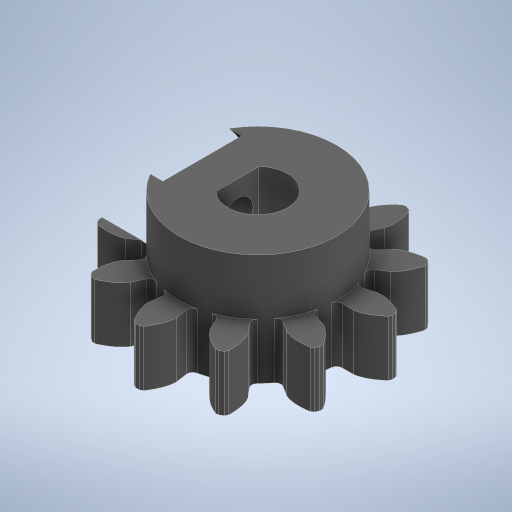
# Autodesk Inventor part: screw_gear_under_12
Saved by Autodesk Inventor 2024.1 (Build 281209000, 209)
## iProperties
Created: 2025-01-10
Part Number: screw_gear_under_12
Material: 一般
Document SubType Name: Modeling
Designer: hibik
Density: 1 g/cm^3
Appearance: 既定
Author: hibik
Autodesk Inventor part; units mm, degrees
ref_plane "XZ Plane" through (0, 0, 0) normal (0, 1, 0) x (-1, 0, 0)
ref_plane "XY Plane" through (0, 0, 0) normal (0, 0, 1) x (1, 0, 0)
sketch "スケッチ1" plane through (0, 0, 0) normal (0, 1, 0) x (-1, 0, 0)
  circle A0 centre (0, 0) radius 5.5 construction
  circle A1 centre (0, 0) radius 5.1683 construction
  line L0 (0, 0) -> (0.7355, -5.1157)
  line L1 (0, -10.5007) -> (0, 8.7501) projected
  dimension "d1" = 10.3366
  dimension "d0" = 11
  dimension "d4" = 8.182
  constraints: 3 coincident, 2 end point, 1 centre point, 7 other
  measures "d0" diameter of A0
  measures "d4" angle of L1 L0
sketch "スケッチ2" plane through (0, 0, 0) normal (0, 1, 0) x (-1, 0, 0)
  circle A0 centre (0, 0) radius 6.5
  dimension "d5" = 13
  constraints: 1 centre point, 1 coincident
  measures "d5" diameter of A0
extrude "押し出し1" add sketch "スケッチ2" along normal blind 3
sketch "スケッチ3" plane through (0, 3, 0) normal (0, 1, 0) x (1, 0, 0)
  line L0 (0, 0) -> (-0.7355, 5.1157) projected
  spline S0 degree 3 poles (-0.7355, 5.1157) (-0.7355, 5.1158) (-0.8126, 5.5427) (-1.3851, 6.0793) (-1.6608, 6.3379) (-2.0474, 6.6147) (-2.557, 6.8472) knots 0 0 0 0 0.674859 0.674859 0.674859 1 1 1 1 projected
  circle A0 centre (0, 0) radius 6.5 projected
  circle A1 centre (0, 0) radius 4.25
  line L1 (0, 10.7) -> (0, -9.95) projected
  point P0 (0, 4.25)
  point P1 (0, 6.5)
  point P2 (-1.6329, 6.2915)
  point P3 (-0.6048, 4.2067)
  dimension "d10" = 8.5
  constraints: 3 coincident, 1 centre point
  measures "d10" diameter of A1
extrude "押し出し2" cut sketch "スケッチ3" against normal through all contours L0 S0 A0 L1 A1 picked at (-0.2452, 5.2886)
fillet "フィレット1" radius 0.3 1 edges at (-0.6048, 1.5, -4.2067)
chamfer "面取り1" distance 0.1 angle 45 1 edges at (-1.6329, 1.5, -6.2915)
mirror "ミラー1" about plane through (0, 3, -6.5) normal (-1, 0, 0) of "押し出し2", "フィレット1", "面取り1"
pattern_circular "円形状パターン1" count 11 over 360 about axis through (0, -10, 0) along (0, 1, 0) of "押し出し2", "フィレット1", "面取り1", "ミラー1"
sketch "スケッチ4" plane through (0, 3, 0) normal (0, 1, 0) x (1, 0, 0)
  circle A0 centre (0, 0) radius 4.25
  dimension "d20" = 8.5
  constraints: 1 centre point, 1 coincident
  measures "d20" diameter of A0
extrude "押し出し3" add sketch "スケッチ4" along normal blind 3
sketch "スケッチ5" plane through (0, 6, 0) normal (0, 1, 0) x (1, 0, 0)
  circle A0 centre (0, 0) radius 1.6
  dimension "d23" = 3.2
  constraints: 1 centre point, 1 coincident
  measures "d23" diameter of A0
extrude "押し出し4" cut sketch "スケッチ5" against normal through all
sketch "スケッチ6" plane through (0, 0, 0) normal (0, -1, 0) x (1, 0, 0)
  circle A0 centre (0, 0) radius 3.05
  dimension "d26" = 6.1
  constraints: 1 centre point, 1 coincident
  measures "d26" diameter of A0
extrude "押し出し5" cut sketch "スケッチ6" against normal blind 2.5
sketch "スケッチ7" plane through (0, 0, 0) normal (1, 0, 0) x (0, 1, 0)
  line L0 (6, -4.25) -> (6, 4.25) projected
  line L1 (2.5, -3.05) -> (2.5, 3.05) projected
  circle A0 centre (4.25, 0) radius 0.85
  line L2 (6, 0) -> (2.5, 0) construction
  point P0 (0, 0)
  dimension "d29" = 1.7
  constraints: 3 midpoint, 2 end point, 1 centre point, 1 coincident, 1 horizontal alignment
  measures "d29" diameter of A0
extrude "押し出し6" cut sketch "スケッチ7" against normal through all
ref_plane "作業平面1" through (-3, 0, 0) normal (1, 0, 0) x (0, 1, 0)
sketch "スケッチ8" plane through (-3, 0, 0) normal (1, 0, 0) x (0, 1, 0)
  circle A0 centre (4.25, 0) radius 2.75
  line L0 (6, 1.6) -> (6, -1.6) projected
  line L1 (2.5, 1.6) -> (2.5, -1.6) projected
  line L2 (2.5, -3.05) -> (2.5, 3.05) projected
  line L3 (6, 0) -> (2.5, 0) construction
  line L4 (2.5, 1.6) -> (2.5, -1.6) projected
  point P0 (0, 0)
  point P1 (2.5, 2.1213)
  point P2 (2.5, -2.1213)
  dimension "d33" = 5.5
  constraints: 3 midpoint, 2 end point, 1 centre point, 1 coincident, 3 other
  measures "d33" diameter of A0
extrude "押し出し7" cut sketch "スケッチ8" against normal through all
ref_plane "作業平面2" through (-1.1, 0, 0) normal (1, 0, 0) x (0, 1, 0)
sketch "スケッチ9" plane through (-1.1, 0, 0) normal (1, 0, 0) x (0, 1, 0)
  line L0 (6, -4.25) -> (6, 4.25) projected
  line L1 (2.5, -3.05) -> (2.5, 3.05) projected
  line L2 (2.5, -1.5) -> (6, -1.5)
  line L3 (6, -1.5) -> (6, 1.5)
  line L4 (6, 1.5) -> (2.5, 1.5)
  line L5 (2.5, 1.5) -> (2.5, -1.5)
  line L6 (2.5, 0) -> (6, 0)
  spline S0 degree 5 poles (5.1, 0) (5.1, 0.1675) (5.0585, 0.3349) (4.9773, 0.4797) (4.8735, 0.5973) (4.664, 0.7501) (4.5679, 0.7993) (4.4647, 0.8329) (4.3574, 0.85) (4.1427, 0.85) (4.0355, 0.8329) (3.9323, 0.7994) (3.8363, 0.7503) (3.6838, 0.6392) (3.6233, 0.5831) (3.5692, 0.5193) (3.5228, 0.4484) (3.4526, 0.3037) (3.4267, 0.2315) (3.4089, 0.1557) (3.4, 0.078) (3.4, -0.1675) (3.4415, -0.3349) (3.5227, -0.4797) (3.6265, -0.5973) (3.836, -0.7501) (3.9321, -0.7993) (4.0353, -0.8329) (4.1426, -0.85) (4.3573, -0.85) (4.4645, -0.8329) (4.5677, -0.7994) (4.6637, -0.7503) (4.8162, -0.6392) (4.8767, -0.5831) (4.9308, -0.5193) (4.9772, -0.4484) (5.0474, -0.3037) (5.0733, -0.2315) (5.0911, -0.1557) (5.1, -0.078) (5.1, 0) knots 0 0 0 0 0 0 0.146408 0.146408 0.146408 0.146408 0.250229 0.250229 0.250229 0.250229 0.353974 0.353974 0.353974 0.353974 0.432259 0.432259 0.432259 0.432259 0.500333 0.500333 0.500333 0.500333 0.646546 0.646546 0.646546 0.646546 0.750229 0.750229 0.750229 0.750229 0.853836 0.853836 0.853836 0.853836 0.932017 0.932017 0.932017 0.932017 1 1 1 1 1 1 projected
  line L7 (2.5, 1.6) -> (2.5, -1.6) projected
  line L8 (6, 1.6) -> (6, -1.6) projected
  point P0 (0, 0)
  point P1 (6, 2.1213)
  point P2 (6, -2.1213)
  point P3 (3, 2.3049)
  point P4 (3, -2.3049)
  point P5 (2.5, 1.5)
  dimension "d37" = 3
  constraints: 10 end point, 3 midpoint, 2 parallel, 2 perpendicular, 1 horizontal, 1 point on line, 5 other
  measures "d37" distance between parallel lines of L4 L2
extrude "押し出し8" add sketch "スケッチ9" against normal up to surface (1.9 mm away) contours L2 L1 L6 S0 L0 | L6 S0 L1 L4 L0
equation "\"module\" = 1"
